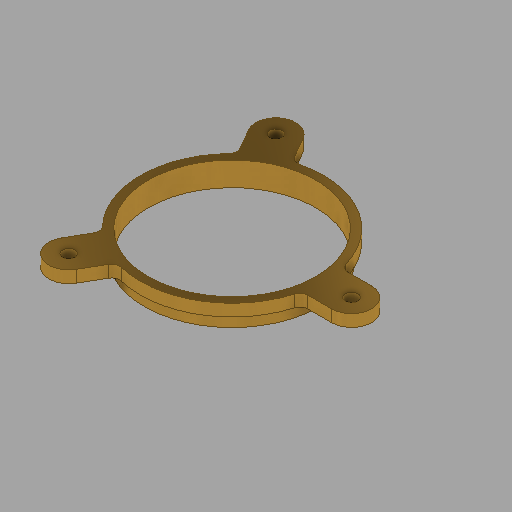
# Autodesk Inventor part: Electrode-Fixed-Press
Saved by Autodesk Inventor 2025 (Build 290162010, 162A)
## iProperties
Created: 2023-08-21
Part Number: Electrode-Fixed-Press
Material: Brass
Document SubType Name: Modeling
Designer: schanen
Density: 8.49 g/cm^3
Appearance: Brass - Polished
Author: schanen
Autodesk Inventor part; units mm, degrees
ref_plane "YZ Plane" through (0, 0, 0) normal (1, 0, 0) x (0, 1, 0)
ref_plane "XZ Plane" through (0, 0, 0) normal (0, 1, 0) x (-1, 0, 0)
ref_plane "XY Plane" through (0, 0, 0) normal (0, 0, 1) x (1, 0, 0)
sketch "Sketch1" plane through (0, 0, 0) normal (0, 0, 1) x (1, 0, 0)
  line L0 (-21, 0) -> (-21, 6)
  line L1 (-21, 6) -> (-23, 6)
  line L2 (-23, 6) -> (-23, 3)
  line L3 (-23, 3) -> (-22, 3)
  line L4 (-22, 3) -> (-22, 0)
  line L5 (-22, 0) -> (-21, 0)
  line L6 (0, -1.2) -> (0, 7.2) projected
  point P0 (0, 0)
  point P1 (-22, 1.5)
  dimension "d0" = 22
  dimension "d1" = 1
  dimension "d2" = 23
  dimension "d3" = 3
  dimension "d4" = 3
  constraints: 12 end point, 5 perpendicular, 1 horizontal alignment, 1 midpoint, 1 vertical
  measures "d0" distance from line of point (0, 0) L4
  measures "d1" distance from line of point (-22, 1.5) L0
  measures "d2" distance between parallel lines of L6 L2
  measures "d3" distance of L3.end L4.end
  measures "d4" distance between parallel lines of L1 L3
revolve "Revolution1" add sketch "Sketch1" angle 360 about axis through (0, -10, 0) along (0, 1, 0)
sketch "Sketch2" plane through (0, 6, 0) normal (0, 1, 0) x (1, 0, 0)
  circle A0 centre (0, 0) radius 30 construction
  circle A1 centre (30, 0) radius 5
  circle A2 centre (0, 0) radius 23 projected
  line L0 (30, 5) -> (22.4499, 5)
  line L1 (30, -5) -> (22.4499, -5)
  dimension "d6" = 60
  dimension "d7" = 10
  constraints: 4 end point, 4 point on circle, 2 horizontal alignment, 2 tangent, 1 centre point, 1 coincident, 1 horizontal, 1 parallel, 2 other
  measures "d7" diameter of A1
extrude "Extrusion1" add sketch "Sketch2" against normal blind 3 contours A1 | A1 L1 A2 L0
fillet "Fillet1" radius 2 2 edges at (22.4499, 4.5, 5) (22.4499, 4.5, -5)
sketch "Sketch3" plane through (30, 6, 0) normal (0, 1, 0) x (1, 0, 0)
  arc A0 (0, -5) -> (0, 5) centre (0, 0) ccw projected
  point P0 (-30, 0)
  constraints: 1 coincident
hole "Hole1" at (30, 6, 0) direction (0, -1, 0) diameter 3.2 end through all clearance for "Flat Head Machine Screw" size "M3" standard "Ansi Metric M Profile"
pattern_circular "Circular Pattern1" count 3 over 360 about axis through (0, 3, 0) along (0, 1, 0) of "Extrusion1", "Hole1", "Fillet1"
body "Solid1"
